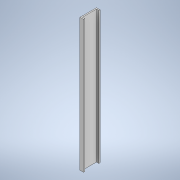
# Autodesk Inventor part: 14in-slide-pt_1
Saved by Autodesk Inventor 2020.1 (Build 241239000, 239)
## iProperties
Created: 2019-09-13
Part Number: 14in-slide-pt_1
Material: Generic
Document SubType Name: Modeling
Designer: alpha
Density: 1 g/cm^3
Appearance: Default
Author: alpha
Autodesk Inventor part; units mm, degrees
ref_plane "YZ Plane" through (0, 0, 0) normal (1, 0, 0) x (0, 1, 0)
ref_plane "XZ Plane" through (0, 0, 0) normal (0, 1, 0) x (-1, 0, 0)
ref_plane "XY Plane" through (0, 0, 0) normal (0, 0, 1) x (1, 0, 0)
sketch "Sketch2" plane through (0, 0, 0) normal (0, 1, 0) x (-1, 0, 0)
  line L0 (-4.7625, -22.225) -> (4.7625, -22.225)
  line L1 (4.7625, -22.225) -> (4.7625, 22.225)
  line L2 (4.7625, 22.225) -> (-4.7625, 22.225)
  line L3 (-4.7625, -22.225) -> (4.7625, 22.225) construction
  line L4 (4.7625, -22.225) -> (-4.7625, 22.225) construction
  line L5 (1.5875, -19.05) -> (1.5875, 19.05)
  line L6 (-11.1125, -19.05) -> (1.5875, 19.05) construction
  line L7 (1.5875, -19.05) -> (-11.1125, 19.05) construction
  line L8 (1.5875, 19.05) -> (-4.7625, 19.05)
  line L9 (1.5875, -19.05) -> (-4.7625, -19.05)
  line L10 (-4.7625, 19.05) -> (-4.7625, 22.225)
  line L11 (-4.7625, -19.05) -> (-4.7625, -22.225)
  point P0 (0, 0)
  point P1 (-4.7625, 0)
  dimension "d0" = 9.525
  dimension "d1" = 44.45
  dimension "d2" = 12.7
  dimension "d3" = 38.1
  constraints: 24 end point, 4 midpoint, 2 vertical, 1 horizontal, 1 parallel, 1 perpendicular
  measures "d0" distance of L2.end L1.end
  measures "d1" distance of L1.end L0.end
  measures "d2" distance of L7.end L5.end
  measures "d3" distance of L5.end L5.start
extrude "Extrusion1" add sketch "Sketch2" along normal blind 355.6
body "Solid1"
